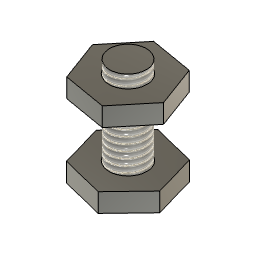
platinum_electrode v46 (Autodesk Fusion 360 archive; units mm, degrees)
design "electrode_bolt"
Autodesk Fusion 360 part; units mm, degrees
sketch "Sketch1" plane through (0, 0, 0) normal (0, 0, 1) x (1, 0, 0)
  circle A0 centre (0, 0) radius 1.5
  dimension "d1" = 3
  constraint coincident A0.centre origin
  measures "d1" diameter of A0
extrude "Extrude1" add sketch "Sketch1" along normal blind 9.5 makes body 1
thread "Thread1" "ISO Metric profile 3.0 M3x0.5 6g" major diameter 2.927 minor diameter 2.3555 pitch 0.5 angle 60 resizes the face on face at (1.4981, -0.0748, 6.3333) on bodies 1
sketch "Sketch2" plane through (0, 0, 9.5) normal (0, 0, 1) x (-1, 0, 0)
  circle A0 centre (0, 0) radius 1.4635
  circle A1 centre (0, 0) radius 1.5
  line L0 (-2.2103, -2.6673) -> (1.2048, -3.2478)
  line L1 (1.2048, -3.2478) -> (3.4151, -0.5805)
  line L2 (3.4151, -0.5805) -> (2.2103, 2.6673)
  line L3 (2.2103, 2.6673) -> (-1.2048, 3.2478)
  line L4 (-1.2048, 3.2478) -> (-3.4151, 0.5805)
  line L5 (-3.4151, 0.5805) -> (-2.2103, -2.6673)
  dimension "d4" = 3
  dimension "d5" = 3
  constraint coincident A0.centre A1.centre
  measures "d4" diameter of A1
  measures "d5" distance of A0.centre L5
extrude "Extrude2" add sketch "Sketch2" against normal blind 2.5 separate body contours L0 L1 L2 L3 L4 L5 makes body 2
extrude "Extrude3" cut 1 faces at (1.9065, -1.6162, 9.5) along direction (0, 0, -1) blind 1 on bodies 2 bodies 2
sketch "Sketch3" plane through (0, 0, 0) normal (0, 0, -1) x (1, 0, 0)
  circle A0 centre (0, 0) radius 1.4635
  line L0 (2.4079, -2.4903) -> (3.3607, 0.8402)
  line L1 (3.3607, 0.8402) -> (0.9527, 3.3305)
  line L2 (0.9527, 3.3305) -> (-2.4079, 2.4903)
  line L3 (-2.4079, 2.4903) -> (-3.3607, -0.8402)
  line L4 (-3.3607, -0.8402) -> (-0.9527, -3.3305)
  line L5 (-0.9527, -3.3305) -> (2.4079, -2.4903)
  circle A1 centre (0, 0) radius 1.5
  dimension "d10" = 3
  dimension "d11" = 3
  constraint coincident A0.centre A1.centre
  measures "d10" distance of A0.centre L5
  measures "d11" diameter of A1
extrude "Extrude4" add sketch "Sketch3" against normal blind 2.5 separate body contours L0 L1 L2 L3 L4 L5 makes body 3
extrude "Extrude5" cut 1 faces at (-1.8043, 1.7303, 0) along direction (0, 0, 1) blind 1 on bodies 3 bodies 3
equation "d2 = 4.5 mm + 1.5 mm + 1.5 mm + 2 mm"
